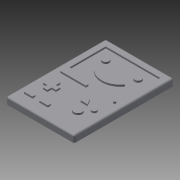
# Autodesk Inventor part: cara
Saved by Autodesk Inventor 2015 (Build 190159000, 159)
## iProperties
Created: 2016-09-11
Part Number: cara
Material: Generic
Document SubType Name: Modeling
Designer: Administrator
Density: 1 g/cm^3
Appearance: Default
Author: Administrator
Autodesk Inventor part; units mm, degrees
ref_plane "YZ Plane" through (0, 0, 0) normal (1, 0, 0) x (0, 1, 0)
ref_plane "XZ Plane" through (0, 0, 0) normal (0, 1, 0) x (-1, 0, 0)
ref_plane "XY Plane" through (0, 0, 0) normal (0, 0, 1) x (1, 0, 0)
sketch "Sketch1" plane through (0, 0, 0) normal (0, 0, 1) x (1, 0, 0)
  line L0 (0, 81.9) -> (0, -81.9) projected
  line L1 (-56, 0) -> (56, 0) projected
  line L2 (-40, 58.5) -> (40, 58.5)
  line L3 (40, 58.5) -> (40, -58.5)
  line L4 (40, -58.5) -> (-40, -58.5)
  line L5 (-40, -58.5) -> (-40, 58.5)
  point P0 (0, 0)
  dimension "d0" = 80
  dimension "d1" = 117
  constraints: 8 end point, 2 parallel, 2 symmetric about line, 1 horizontal, 1 perpendicular
  measures "d0" distance of L3.end L4.end
  measures "d1" distance of L2.end L3.end
extrude "Extrusion1" add sketch "Sketch1" along normal blind 8
sketch "Sketch2" plane through (0, 0, 8) normal (0, 0, 1) x (1, 0, 0)
  line L0 (40, 58.5) -> (-40, 58.5) projected
  line L1 (-40, 58.5) -> (-40, -58.5) projected
  line L2 (-40, -58.5) -> (40, -58.5) projected
  line L3 (40, -58.5) -> (40, 58.5) projected
  line L4 (-56, 0) -> (56, 0) projected
  line L5 (0, -81.9) -> (0, 81.9) projected
  line L6 (-32, 0) -> (-1.8784, 0)
  line L7 (-1.8784, 0) -> (-1.8784, -3)
  line L8 (-1.8784, -3) -> (-32, -3)
  line L9 (-32, -3) -> (-32, 0)
  line L10 (-25, -15) -> (-25, -20)
  line L11 (-25, -20) -> (-30, -20)
  line L12 (-30, -20) -> (-30, -25)
  line L13 (-30, -25) -> (-25, -25)
  line L14 (-25, -25) -> (-25, -30)
  line L15 (-25, -30) -> (-20, -30)
  line L16 (-20, -30) -> (-20, -25)
  line L17 (-20, -25) -> (-15, -25)
  line L18 (-15, -25) -> (-15, -20)
  line L19 (-15, -20) -> (-20, -20)
  line L20 (-20, -20) -> (-20, -15)
  line L21 (-20, -15) -> (-25, -15)
  line L22 (14, -14) -> (10, -20.9282)
  line L23 (10, -20.9282) -> (18, -20.9282)
  circle A0 centre (27, -22) radius 3
  circle A1 centre (18, -32) radius 5
  line L24 (-32, -42) -> (-22, -42)
  line L25 (-22, -42) -> (-22, -45.5)
  line L26 (-22, -45.5) -> (-32, -45.5)
  line L27 (-32, -45.5) -> (-32, -42)
  line L28 (-14, -42) -> (-4, -42)
  line L29 (-4, -42) -> (-4, -45.5)
  line L30 (-4, -45.5) -> (-14, -45.5)
  line L31 (-14, -45.5) -> (-14, -42)
  circle A2 centre (30.5, -1.5) radius 1.5
  line L32 (14, -20.9282) -> (14, -9.9927) construction
  line L33 (14, -14) -> (18, -20.9282)
  line L34 (-1.8784, -1.5) -> (30.5, -1.5) construction
  line L35 (-32, 50.5) -> (32, 50.5) construction
  line L36 (32, 50.5) -> (32, 8) construction
  line L37 (32, 8) -> (-32, 8) construction
  line L38 (-32, 8) -> (-32, 50.5) construction
  point P0 (0, 0)
  dimension "d4" = 3
  dimension "d5" = 8
  dimension "d7" = 5
  dimension "d8" = 60
  dimension "d9" = 10
  dimension "d10" = 12
  dimension "d11" = 12
  dimension "d12" = 3
  dimension "d13" = 8
  dimension "d14" = 8
  dimension "d15" = 8
  dimension "d16" = 10
  dimension "d17" = 22
  dimension "d18" = 22
  dimension "d19" = 22
  dimension "d20" = 40
  dimension "d21" = 30
  dimension "d22" = 13
  dimension "d23" = 6
  dimension "d24" = 10
  dimension "d25" = 13
  dimension "d26" = 8
  constraints: 66 end point, 12 perpendicular, 10 point on line, 6 equal length, 6 horizontal, 5 parallel, 3 centre point, 3 collinear, 2 midpoint, 2 vertical, 1 coincident, 1 symmetric about line, 1 tangent
  measures "d4" distance of L6.end L7.end
  measures "d5" distance of L22.end L23.end
  measures "d7" distance of L10.end L11.end
  measures "d8" angle of L22 L23
  measures "d9" distance between parallel lines of L1 L12
  measures "d10" distance between parallel lines of L21 L8
  measures "d11" distance between parallel lines of L24 L15
  measures "d12" diameter of A2
  measures "d13" distance between parallel lines of L0 L35
  measures "d14" distance between parallel lines of L1 L38
  measures "d15" distance from line of L37.end L4
  measures "d16" diameter of A1
  measures "d17" distance from line of L3 L23.end
  measures "d18" distance from line of L37 L22.start
  measures "d19" distance from line of L3 A1.centre
  measures "d20" distance from line of A1.centre L37
  measures "d21" distance from line of A0.centre L37
  measures "d22" distance from line of L3 A0.centre
  measures "d23" diameter of A0
  measures "d24" distance of L25.end L26.end
  measures "d25" distance from line of L2 L26.end
  measures "d26" distance between parallel lines of L31 L25
extrude "Extrusion2" add sketch "Sketch2" along normal blind 2 contours A2 | L7 L8 L9 L4 | L21 L20 L19 L18 L17 L16 L15 L14 L13 L12 L11 L10 | L33 L23 L22 | A0 | A1 | L24 L25 L26 L27 | L28 L29 L30 L31
sketch "Sketch3" plane through (0, 0, 8) normal (0, 0, 1) x (1, 0, 0)
  line L0 (-32, 0) -> (-1.8784, 0) projected
  line L1 (-1.8784, 0) -> (-1.8784, -3) projected
  line L2 (-1.8784, -3) -> (-32, -3) projected
  line L3 (-32, -3) -> (-32, 0) projected
  line L4 (-4, -42) -> (-4, -45.5) projected
  line L5 (-4, -45.5) -> (-14, -45.5) projected
  line L6 (-14, -45.5) -> (-14, -42) projected
  line L7 (-14, -42) -> (-4, -42) projected
  circle A0 centre (27, -22) radius 3 projected
  circle A1 centre (30.5, -1.5) radius 1.5 projected
  line L8 (14, -14) -> (18, -20.9282) projected
  line L9 (18, -20.9282) -> (10, -20.9282) projected
  line L10 (10, -20.9282) -> (14, -14) projected
  line L11 (-22, -42) -> (-22, -45.5) projected
  line L12 (-22, -45.5) -> (-32, -45.5) projected
  line L13 (-32, -45.5) -> (-32, -42) projected
  line L14 (-32, -42) -> (-22, -42) projected
  circle A2 centre (18, -32) radius 5 projected
  line L15 (-25, -15) -> (-20, -15) projected
  line L16 (-20, -15) -> (-20, -20) projected
  line L17 (-20, -20) -> (-15, -20) projected
  line L18 (-15, -20) -> (-15, -25) projected
  line L19 (-15, -25) -> (-20, -25) projected
  line L20 (-20, -25) -> (-20, -30) projected
  line L21 (-20, -30) -> (-25, -30) projected
  line L22 (-25, -30) -> (-25, -25) projected
  line L23 (-25, -25) -> (-30, -25) projected
  line L24 (-30, -25) -> (-30, -20) projected
  line L25 (-30, -20) -> (-25, -20) projected
  line L26 (-25, -20) -> (-25, -15) projected
  line L27 (40, 58.5) -> (-40, 58.5) projected
  line L28 (-40, 58.5) -> (-40, -58.5) projected
  line L29 (-40, -58.5) -> (40, -58.5) projected
  line L30 (40, -58.5) -> (40, 58.5) projected
  line L31 (-32, 50.5) -> (32, 50.5)
  line L32 (32, 50.5) -> (32, 8)
  line L33 (32, 8) -> (-32, 8)
  line L34 (-32, 8) -> (-32, 50.5)
  line L35 (-56, 0) -> (56, 0) projected
  line L36 (0, -81.9) -> (0, 81.9) projected
  point P0 (0, 0)
  dimension "d29" = 8
  dimension "d30" = 8
  dimension "d31" = 8
  constraints: 8 end point, 2 parallel, 1 horizontal, 1 perpendicular, 1 symmetric about line
  measures "d29" distance between parallel lines of L31 L27
  measures "d30" distance between parallel lines of L33 L35
  measures "d31" distance between parallel lines of L28 L34
extrude "Extrusion3" cut sketch "Sketch3" against normal blind 2 contours L36 L31 L32 L33 | L33 L34 L31 L36
sketch "Sketch4" plane through (0, 0, 6) normal (0, 0, 1) x (1, 0, 0)
  line L0 (-32, 50.5) -> (32, 50.5) projected
  line L1 (-32, 8) -> (-32, 50.5) projected
  line L2 (32, 8) -> (-32, 8) projected
  line L3 (32, 50.5) -> (32, 8) projected
  line L4 (32, 50.5) -> (32, 8) projected
  arc A0 (-16.4483, 24.1223) -> (16.4483, 24.1223) centre (0, 35.5) ccw
  arc A1 (-17.9287, 23.0983) -> (17.9287, 23.0983) centre (0, 35.5) ccw
  line L5 (-17.9287, 23.0983) -> (-16.4483, 24.1223)
  line L6 (16.4483, 24.1223) -> (17.9287, 23.0983)
  line L7 (-56, 0) -> (56, 0) projected
  line L8 (0, -81.9) -> (0, 81.9) projected
  circle A2 centre (-19, 37.5) radius 4
  circle A3 centre (19, 37.5) radius 4
  point P0 (0, 0)
  dimension "d36" = 1.8
  dimension "d41" = 20
  dimension "d42" = 15
  dimension "d43" = 1.024
  dimension "d44" = 8
  dimension "d45" = 13
  dimension "d46" = 13
  constraints: 4 centre point, 4 end point, 4 point on circle, 1 point on line, 1 symmetric about line, 1 other
  measures "d36" radial gap between concentric circles of A1 A0
  measures "d41" radius of A0
  measures "d42" distance from line of A0.centre L0
  measures "d43" vertical distance of L6.start L6.end
  measures "d44" diameter of A2
  measures "d45" distance from line of L1 A2.centre
  measures "d46" distance from line of L0 A2.centre
extrude "Extrusion6" add sketch "Sketch4" along normal blind 2 contours L8 A1 L5 A0 | A0 L6 A1 L8 | A2 | A3
fillet "Fillet1" [suppressed]
sketch "Sketch5" plane through (0, 0, 0) normal (0, 0, -1) x (-1, 0, 0)
  line L0 (40, 58.5) -> (-40, 58.5) projected
  line L1 (-40, 58.5) -> (-40, -58.5) projected
  line L2 (-40, -58.5) -> (40, -58.5) projected
  line L3 (40, -58.5) -> (40, 58.5) projected
  circle A0 centre (-35, 53.5) radius 2.75
  line L4 (56, 0) -> (-56, 0) projected
  line L5 (0, -81.9) -> (0, 81.9) projected
  circle A1 centre (35, 53.5) radius 2.75
  circle A2 centre (-35, -53.5) radius 2.75
  circle A3 centre (35, -53.5) radius 2.75
  point P0 (0, 0)
  dimension "d51" = 5.5
  dimension "d52" = 5
  dimension "d53" = 5
  constraints: 4 centre point, 3 symmetric about line, 3 other
  measures "d51" diameter of A0
  measures "d52" distance from line of L0 A0.centre
  measures "d53" distance from line of L1 A0.centre
extrude "Extrusion7" cut sketch "Sketch5" against normal blind 4 contours A0 | A1 | A2 | A3
fillet "Fillet2" radius 2 8 edges at (0, 58.5, 8) (40, 58.5, 4) (40, 0, 8) (-40, 58.5, 4) (-40, 0, 8) (40, -58.5, 4) (0, -58.5, 8) (-40, -58.5, 4)
fillet "Fillet3" radius 0.8 4 edges at (37.75, -53.5, 0) (-32.25, -53.5, 0) (37.75, 53.5, 0) (-32.25, 53.5, 0)
equation "\"d12\" = d4"
equation "\"d14\" = d13"
body "Solid1"
